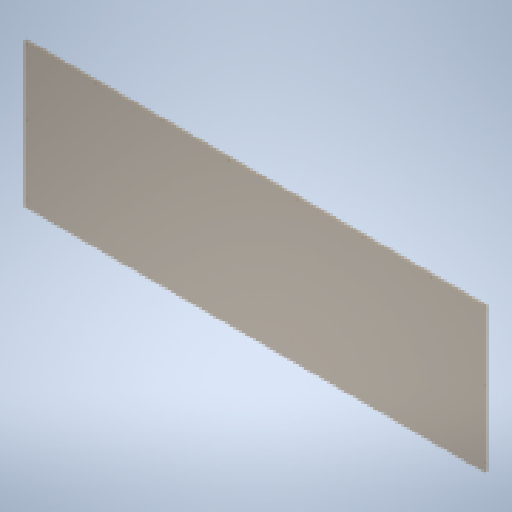
# Autodesk Inventor part: Polycarb
Saved by Autodesk Inventor 2024 (Build 280153000, 153)
## iProperties
Created: 2023-04-16
Part Number: Polycarb
Material: Polycarbonate, Smoke
Document SubType Name: Modeling
Designer: legom
Density: 1.2 g/cm^3
Appearance: Polycarbonate - Smoked
Author: legom
Autodesk Inventor part; units mm, degrees
ref_plane "YZ Plane" through (0, 0, 0) normal (1, 0, 0) x (0, 1, 0)
ref_plane "XZ Plane" through (0, 0, 0) normal (0, 1, 0) x (-1, 0, 0)
ref_plane "XY Plane" through (0, 0, 0) normal (0, 0, 1) x (1, 0, 0)
sketch "Sketch1" plane through (0, 0, 0) normal (0, 0, 1) x (1, 0, 0)
  line L0 (-1124.9025, 458.1525) -> (1313.4975, 458.1525)
  line L1 (1313.4975, 458.1525) -> (1313.4975, -303.8475)
  line L2 (1313.4975, -303.8475) -> (-1124.9025, -303.8475)
  line L3 (-1124.9025, -303.8475) -> (-1124.9025, 458.1525)
  point P0 (0, 0)
  dimension "d0" = 2438.4
  dimension "d1" = 762
  constraints: 8 end point, 2 parallel, 1 horizontal, 1 perpendicular
  measures "d0" distance of L0.start L0.end
  measures "d1" distance of L0.end L1.end
extrude "Extrusion1" add sketch "Sketch1" along normal blind 12.7
sketch "Sketch2" plane through (0, 0, 12.7) normal (0, 0, 1) x (1, 0, 0)
  circle A0 centre (-1112.2025, 445.4525) radius 2.5527
  line L0 (1313.4975, 458.1525) -> (-1124.9025, 458.1525) projected
  line L1 (-1124.9025, 458.1525) -> (-1124.9025, -303.8475) projected
  point P0 (0, 0)
  dimension "d4" = 5.1054
  dimension "d5" = 12.7
  dimension "d6" = 12.7
  constraints: 1 centre point
  measures "d4" diameter of A0
  measures "d5" distance from line of L0 A0.centre
  measures "d6" distance from line of L1 A0.centre
extrude "Extrusion2" cut sketch "Sketch2" against normal through all
pattern_linear "Rectangular Pattern1" count 3 spacing 355.6 along (0, -1, 0) of "Extrusion2"
pattern_linear "Rectangular Pattern2" count 8 spacing 355.6 along (1, 0, 0) of "Extrusion2"
pattern_linear "Rectangular Pattern3" count 2 spacing 2413 along (1, 0, 0) of "Extrusion2", "Rectangular Pattern1"
body "Solid1"
